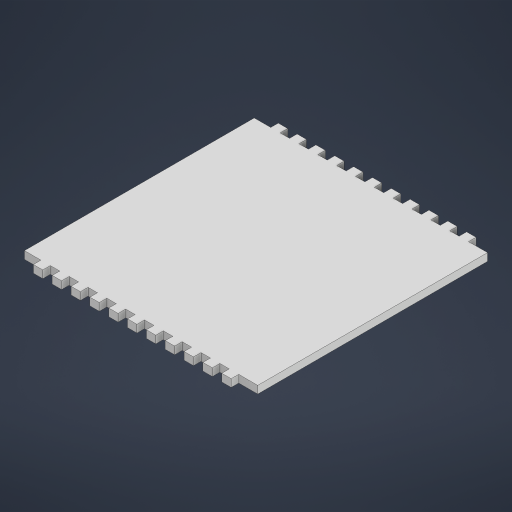
# Autodesk Inventor part: ZwischenEbene
Saved by Autodesk Inventor 2023 (Build 270158030, 158C)
## iProperties
Created: 2022-06-23
Part Number: ZwischenEbene
Material: Generic
Document SubType Name: Modeling
Designer: Simon
Density: 1 g/cm^3
Appearance: Default
Author: Simon
Autodesk Inventor part; units mm, degrees
ref_plane "YZ Plane" through (0, 0, 0) normal (1, 0, 0) x (0, 1, 0)
ref_plane "XZ Plane" through (0, 0, 0) normal (0, 1, 0) x (-1, 0, 0)
ref_plane "XY Plane" through (0, 0, 0) normal (0, 0, 1) x (1, 0, 0)
sketch "Sketch1" plane through (0, 0, 0) normal (0, 1, 0) x (-1, 0, 0)
  line L0 (-80.0987, 126) -> (-80.0987, 4)
  line L1 (-75.0987, 4) -> (-80.0987, 4)
  line L2 (-75.0987, 4) -> (-70.0987, 4)
  line L3 (-70, 0) -> (-70, 4)
  line L4 (-65, 0) -> (-70, 0)
  line L5 (-65, 0) -> (-65, 4)
  line L6 (43.75, 4) -> (-80.0987, 4)
  line L7 (-60, 0) -> (-60, 4)
  line L8 (-55, 0) -> (-55, 4)
  line L9 (-50, 0) -> (-50, 4)
  line L10 (-45, 0) -> (-45, 4)
  line L11 (-35, 0) -> (-35, 4)
  line L12 (-40, 0) -> (-40, 4)
  line L13 (-30, 0) -> (-30, 4)
  line L14 (-25, 0) -> (-25, 4)
  line L15 (-20, 0) -> (-20, 4)
  line L16 (-15, 0) -> (-15, 4)
  line L17 (-10, 0) -> (-10, 4)
  line L18 (-5, 0) -> (-5, 4)
  line L19 (0, 0) -> (0, 4)
  line L20 (5, 0) -> (5, 4)
  line L21 (10, 0) -> (10, 4)
  line L22 (15, 0) -> (15, 4)
  line L23 (20, 0) -> (20, 4)
  line L24 (25, 0) -> (25, 4)
  line L25 (30, 0) -> (30, 4)
  line L26 (35, 0) -> (35, 4)
  line L27 (43.75, 126) -> (43.75, 4)
  line L28 (43.75, 126) -> (-80.0987, 126)
  line L29 (-70, 126) -> (-70, 130)
  line L30 (-70, 130) -> (-65, 130)
  line L31 (-65, 126) -> (-65, 130)
  line L32 (-60, 126) -> (-60, 130)
  line L33 (-60, 130) -> (-55, 130)
  line L34 (-55, 126) -> (-55, 130)
  line L35 (-50, 126) -> (-50, 130)
  line L36 (-50, 130) -> (-45, 130)
  line L37 (-45, 126) -> (-45, 130)
  line L38 (-40, 126) -> (-40, 130)
  line L39 (-40, 130) -> (-35, 130)
  line L40 (-35, 126) -> (-35, 130)
  line L41 (-30, 126) -> (-30, 130)
  line L42 (-30, 130) -> (-25, 130)
  line L43 (-25, 126) -> (-25, 130)
  line L44 (-20, 126) -> (-20, 130)
  line L45 (-20, 130) -> (-15, 130)
  line L46 (-15, 126) -> (-15, 130)
  line L47 (-10, 126) -> (-10, 130)
  line L48 (-10, 130) -> (-5, 130)
  line L49 (-5, 126) -> (-5, 130)
  line L50 (0, 130) -> (5, 130)
  line L51 (5, 126) -> (5, 130)
  line L52 (0, 126) -> (0, 130)
  line L53 (10, 126) -> (10, 130)
  line L54 (10, 130) -> (15, 130)
  line L55 (15, 126) -> (15, 130)
  line L56 (20, 126) -> (20, 130)
  line L57 (20, 130) -> (25, 130)
  line L58 (25, 126) -> (25, 130)
  line L59 (30, 126) -> (30, 130)
  line L60 (30, 130) -> (35, 130)
  line L61 (35, 126) -> (35, 130)
  line L62 (35, 0) -> (30, 0)
  line L63 (25, 0) -> (20, 0)
  line L64 (15, 0) -> (10, 0)
  line L65 (5, 0) -> (0, 0)
  line L66 (-5, 0) -> (-10, 0)
  line L67 (-15, 0) -> (-20, 0)
  line L68 (-25, 0) -> (-30, 0)
  line L69 (-35, 0) -> (-40, 0)
  line L70 (-45, 0) -> (-50, 0)
  line L71 (-55, 0) -> (-60, 0)
  line L72 (-65, 0) -> (-70, 0)
  constraints: 142 end point, 10 collinear, 3 horizontal, 1 vertical, 7 other
extrude "Extrusion1" add sketch "Sketch1" along normal blind 4
body "Solid1"
